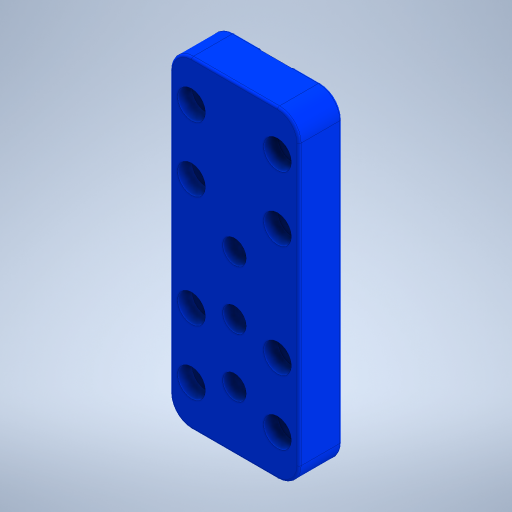
# Autodesk Inventor part: AdapterLinearGuideLong
Saved by Autodesk Inventor 2024 (Build 280153000, 153)
## iProperties
Created: 2023-12-27
Part Number: AdapterLinearGuideLong
Material: Generisch
Document SubType Name: Modeling
Designer: denni
Density: 1 g/cm^3
Appearance: Vorgabe(2)
Author: denni
Autodesk Inventor part; units mm, degrees
ref_plane "YZ Plane" through (0, 0, 0) normal (1, 0, 0) x (0, 1, 0)
ref_plane "XZ Plane" through (0, 0, 0) normal (0, 1, 0) x (-1, 0, 0)
ref_plane "XY Plane" through (0, 0, 0) normal (0, 0, 1) x (1, 0, 0)
sketch "Skizze1" plane through (0, 0, 0) normal (0, 0, 1) x (1, 0, 0)
  line L0 (0, 0) -> (30, 0)
  line L1 (30, 0) -> (30, 75)
  line L2 (30, 75) -> (0, 75)
  line L3 (0, 75) -> (0, 0)
  dimension "d0" = 30
  dimension "d1" = 75
  constraints: 8 end point, 2 parallel, 1 horizontal, 1 perpendicular
  measures "d0" distance of L1.end L2.end
  measures "d1" distance of L2.end L0.start
extrude "Extrusion1" add sketch "Skizze1" along normal blind 10
sketch "Skizze2" plane through (0, 0, 10) normal (0, 0, 1) x (1, 0, 0)
  line L0 (5, 65.5) -> (25, 65.5) construction
  line L1 (25, 65.5) -> (25, 50.5) construction
  line L2 (25, 50.5) -> (5, 50.5) construction
  line L3 (5, 50.5) -> (5, 65.5) construction
  line L4 (5, 9.5) -> (25, 9.5) construction
  line L5 (25, 9.5) -> (25, 24.5) construction
  line L6 (25, 24.5) -> (5, 24.5) construction
  line L7 (5, 24.5) -> (5, 9.5) construction
  line L8 (30, 75) -> (0, 75) construction
  line L9 (0, 0) -> (30, 0) construction
  line L10 (15, 65.5) -> (15, 75) construction
  line L11 (15, 50.5) -> (15, 24.5) construction
  dimension "d4" = 9.5
  dimension "d5" = 15
  dimension "d6" = 9.5
  dimension "d7" = 15
  dimension "d8" = 20
  constraints: 20 end point, 8 coincident, 4 midpoint, 4 parallel, 3 perpendicular, 2 horizontal, 2 point on line
  measures "d4" distance between parallel lines of L8 L0
  measures "d5" distance of L2.end L0.start
  measures "d6" distance between parallel lines of L9 L4
  measures "d7" distance of L6.end L4.start
  measures "d8" distance of L0.start L0.end
hole "Bohrung1" at (5, 65.5, 10) at (25, 65.5, 10) at (25, 50.5, 10) at (5, 50.5, 10) at (5, 24.5, 10) at (25, 24.5, 10) at (25, 9.5, 10) at (5, 9.5, 10) direction (0, 0, -1) diameter 3.4 end through all counterbore diameter 6.5 counterbore depth 3.4 clearance for "Inbusschraube ISO 4762" size "M3" standard "ISO"
sketch "Skizze4" plane through (0, 0, 0) normal (0, 0, -1) x (-1, 0, 0)
  line L0 (-18.5, 75) -> (-11.5, 75)
  line L1 (-11.5, 75) -> (-11.5, 55)
  line L2 (-11.5, 55) -> (-18.5, 55)
  line L3 (-18.5, 55) -> (-18.5, 75)
  line L4 (-30, 75) -> (0, 75) projected
  point P0 (0, 0)
  point P1 (-15, 75)
  dimension "d22" = 20
  dimension "d23" = 7
  constraints: 8 end point, 2 midpoint, 2 parallel, 1 horizontal, 1 perpendicular
  measures "d22" distance of L2.end L0.start
  measures "d23" distance of L1.end L2.end
extrude "Extrusion3" cut sketch "Skizze4" against normal blind 0.5
fillet "Rundung1" radius 5 4 edges at (0, 75, 5) (30, 75, 5) (0, 0, 5) (30, 0, 5)
fillet "Rundung3" radius 0.5 4 edges at (18.5, 75, 0.25) (11.5, 75, 0.25) (18.5, 55, 0.25) (11.5, 55, 0.25)
fillet "Rundung2" radius 0.5 24 edges at (1.4645, 73.5355, 10) (0, 37.5, 10) (1.4645, 1.4645, 10) (15, 0, 10) (28.5355, 1.4645, 10) (30, 37.5, 10) (28.5355, 73.5355, 10) (15, 75, 10) (18.6464, 74.8536, 0) (18.5, 65, 0) (18.3536, 55.1464, 0) (15, 55, 0) (11.6464, 55.1464, 0) (11.5, 65, 0) (11.3536, 74.8536, 0) (8, 75, 0) (1.4645, 73.5355, 0) (0, 37.5, 0) (1.4645, 1.4645, 0) (15, 0, 0) (28.5355, 1.4645, 0) (30, 37.5, 0) (28.5355, 73.5355, 0) (22, 75, 0)
sketch "Skizze5" plane through (0, 0, 0) normal (0, 0, -1) x (-1, 0, 0)
  line L0 (-18, 54.5) -> (-12, 54.5) construction
  line L1 (-15, 54.5) -> (-15, 40.875) construction
  line L2 (-15, 40.875) -> (-15, 27.25) construction
  line L3 (-15, 27.25) -> (-15, 13.625) construction
  line L4 (-15, 13.625) -> (-15, 0) construction
  line L5 (-5, 0) -> (-25, 0) construction
  point P0 (0, 0)
  constraints: 8 end point, 5 collinear, 3 coincident, 2 midpoint, 1 perpendicular
hole "Bohrung2" at (15, 13.625, 0) at (15, 27.25, 0) at (15, 40.875, 0) direction (0, 0, 1) diameter 5.5 end through all counterbore diameter 10 counterbore depth 5.7 clearance for "Inbusschraube ISO 4762" size "M5" standard "ISO"
